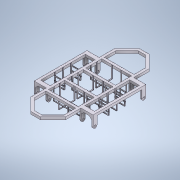
# Autodesk Inventor part: Rahmen_neu
Saved by Autodesk Inventor 2020 (Build 240168000, 168)
## iProperties
Created: 2020-04-28
Part Number: Rahmen_neu
Material: Aluminum 6061, geschweißt
Document SubType Name: Modeling
Designer: Chris
Density: 2.7 g/cm^3
Appearance: Schweißnaht - Aluminum
Mass: 36293.4 g
Surface Area: 46389.4 cm^2
Volume: 13442 cm^3
Author: Chris
Autodesk Inventor part; units mm, degrees
ref_plane "YZ Plane" through (0, 0, 0) normal (1, 0, 0) x (0, 1, 0)
ref_plane "XZ Plane" through (0, 0, 0) normal (0, 1, 0) x (-1, 0, 0)
ref_plane "XY Plane" through (0, 0, 0) normal (0, 0, 1) x (1, 0, 0)
sketch "Skizze1" plane through (0, 0, 0) normal (0, 1, 0) x (-1, 0, 0)
  line L0 (0, 0) -> (590, 0)
  line L1 (590, 0) -> (590, -1060)
  line L2 (590, -1060) -> (0, -1060)
  line L3 (0, -1060) -> (0, 0)
  line L4 (0, 0) -> (-50, 0)
  line L5 (-50, 0) -> (-50, 50)
  line L6 (-50, 50) -> (0, 50)
  line L7 (0, 50) -> (0, 0)
  line L8 (-50, 50) -> (640, 50)
  line L9 (640, 50) -> (640, -1110)
  line L10 (640, -1110) -> (-50, -1110)
  line L11 (-50, -1110) -> (-50, 50)
  line L12 (590, 0) -> (590, -320) construction
  line L13 (590, -320) -> (590, -370) construction
  line L14 (590, -370) -> (590, -690) construction
  line L15 (590, -690) -> (590, -740) construction
  line L16 (590, -740) -> (590, -1060) construction
  line L17 (590, -320) -> (0, -320)
  line L18 (590, -370) -> (0, -370)
  line L19 (590, -690) -> (0, -690)
  line L20 (590, -740) -> (0, -740)
  dimension "d0" = 590
  dimension "d1" = 1060
  dimension "d3" = 50
  dimension "d4" = 50
  dimension "d5" = 690
  dimension "d6" = 1160
  dimension "d38" = 320
  dimension "d39" = 50
  dimension "d40" = 320
  dimension "d41" = 50
  dimension "d42" = 320
  constraints: 42 end point, 8 point on line, 7 perpendicular, 6 parallel, 3 horizontal, 1 collinear
  measures "d0" distance of L1.end L2.end
  measures "d1" distance of L0.end L1.end
  measures "d3" distance of L5.end L6.end
  measures "d4" distance of L4.end L5.end
  measures "d5" distance of L9.end L10.end
  measures "d6" distance of L8.end L9.end
  measures "d38" distance of L0.end L12.end
  measures "d39" distance of L12.end L13.end
  measures "d40" distance of L13.end L14.end
  measures "d41" distance of L14.end L15.end
  measures "d42" distance of L15.end L1.end
extrude "Extrusion1" add sketch "Skizze1" along normal blind 50 contours L7 L8 L9 L10 L11 L4 | L4 L5 L6 L7 | L17 L1 L18 L3 | L19 L1 L20 L3
sketch "Skizze2" plane through (0, 50, 0) normal (0, 1, 0) x (1, 0, 0)
  line L0 (-640, -50) -> (50, -50) projected
  line L1 (-640, -50) -> (-380, -50) construction
  line L2 (50, -300) -> (50, -50)
  line L3 (50, -300) -> (-200, -550)
  line L4 (50, -300) -> (403.5534, -300) construction
  line L5 (-220.7107, -500) -> (0.0003, -279.289)
  line L6 (0.0003, -279.289) -> (0.0003, -50)
  line L7 (-630, 530) -> (45, 530) construction
  line L8 (-640, -50) -> (-640, -550) construction
  line L9 (-640, -50) -> (-140, -50) construction
  line L10 (-640, -50) -> (-640, -300)
  line L11 (-640, -300) -> (-390, -550)
  line L12 (-390, -550) -> (-200, -550)
  line L13 (-515, -425) -> (-479.6447, -389.6447) construction
  line L14 (-640, -50) -> (50, -50) projected
  line L15 (-590, -50) -> (-590, -279.2893)
  line L16 (-590, -279.2893) -> (-369.2893, -500)
  line L17 (-369.2893, -500) -> (-220.7107, -500)
  line L18 (-640, -50) -> (-590, -50)
  line L19 (0.0003, -50) -> (50, -50)
  line L20 (-640, 1110) -> (50, 1110)
  line L21 (-640, 1110) -> (-380, 1110) construction
  line L22 (50, 1360) -> (50, 1110)
  line L23 (50, 1360) -> (-200, 1610)
  line L24 (50, 1360) -> (403.5534, 1360) construction
  line L25 (-220.7107, 1560) -> (0.0003, 1339.289)
  line L26 (0.0003, 1339.289) -> (0.0003, 1110)
  line L27 (-640, 1110) -> (-640, 1610) construction
  line L28 (-640, 1110) -> (-140, 1110) construction
  line L29 (-640, 1110) -> (-640, 1360)
  line L30 (-640, 1360) -> (-390, 1610)
  line L31 (-390, 1610) -> (-200, 1610)
  line L32 (-515, 1485) -> (-479.6447, 1449.6447) construction
  line L33 (-640, 1110) -> (50, 1110)
  line L34 (-590, 1110) -> (-590, 1339.2893)
  line L35 (-590, 1339.2893) -> (-369.2893, 1560)
  line L36 (-369.2893, 1560) -> (-220.7107, 1560)
  line L37 (-640, 1110) -> (-590, 1110)
  line L38 (0.0003, 1110) -> (50, 1110)
  point P0 (0, 0)
  point P1 (-640, 1110)
  point P2 (50, 1110)
  point P3 (0, 1060)
  dimension "d13" = 250
  dimension "d14" = 90
  dimension "d28" = 135
  dimension "d32" = 50
  dimension "d33" = 220.711
  dimension "d81" = 500
  dimension "d82" = 90
  dimension "d83" = 250
  dimension "d84" = 135
  dimension "d87" = 50
  dimension "d88" = 50
  dimension "d89" = 50
  constraints: 74 end point, 21 symmetric about line, 5 horizontal, 4 point on line, 3 midpoint, 3 perpendicular, 2 equal length, 1 collinear, 1 vertical
  measures "d13" distance of L2.start L0.end
  measures "d14" angle of L2 L0
  measures "d28" angle of L3 L4
  measures "d32" distance between parallel lines of L3 L5
  measures "d33" horizontal distance of L5.start L5.end
  measures "d81" distance of L0.start L8.end
  measures "d82" angle of L8 L9
  measures "d83" distance of L0.start L10.end
  measures "d84" angle of L11 L10
  measures "d87" distance of L13.start L13.end
  measures "d88" distance between parallel lines of L12 L17
  measures "d89" distance between parallel lines of L15 L8
extrude "Extrusion2" add sketch "Skizze2" against normal blind 50 contours L0 L15 L16 L17 L5 L6 L2 L3 L12 L11 L10 | L29 L30 L31 L23 L22 L20 L26 L25 L36 L35 L34
sketch "Skizze3" plane through (0, 50, 0) normal (0, 1, 0) x (1, 0, 0)
  line L0 (-590, 370) -> (-590, 690) construction
  line L1 (-634.8333, 530) -> (-634.8333, 1015) construction
  line L2 (-640, 1360) -> (-640, -300) construction
  line L3 (-200, -550) -> (-380, -550) construction
  line L4 (-380, 1610) -> (-200, 1610) construction
  line L5 (-640, 530) -> (-640, 45) construction
  line L6 (-640, 45) -> (-880, 45)
  line L7 (-880, 45) -> (-880, 85)
  line L8 (-880, 85) -> (-640, 85)
  line L9 (-640, 85) -> (-640, 45)
  line L10 (-640, 45) -> (-880, 45)
  line L11 (-880, 45) -> (-880, 5)
  line L12 (-880, 5) -> (-640, 5)
  line L13 (-640, 5) -> (-640, 45)
  line L14 (50, -300) -> (50, 1360) projected
  line L15 (50, 530) -> (-640, 530)
  line L16 (-390, -550) -> (-200, -550) projected
  line L17 (-295, -550) -> (-295, 1610)
  line L18 (-390, 1610) -> (-200, 1610) projected
  line L19 (50, 45) -> (290, 45)
  line L20 (290, 45) -> (290, 85)
  line L21 (290, 85) -> (50, 85)
  line L22 (50, 85) -> (50, 45)
  line L23 (50, 45) -> (290, 45)
  line L24 (290, 45) -> (290, 5)
  line L25 (290, 5) -> (50, 5)
  line L26 (50, 5) -> (50, 45)
  line L27 (-640, 1015) -> (-880, 1015)
  line L28 (-880, 1015) -> (-880, 975)
  line L29 (-880, 975) -> (-640, 975)
  line L30 (-640, 975) -> (-640, 1015)
  line L31 (-640, 1015) -> (-880, 1015)
  line L32 (-880, 1015) -> (-880, 1055)
  line L33 (-880, 1055) -> (-640, 1055)
  line L34 (-640, 1055) -> (-640, 1015)
  line L35 (50, 975) -> (50, 1015)
  line L36 (50, 1055) -> (50, 1015)
  line L37 (290, 1015) -> (290, 975)
  line L38 (290, 975) -> (50, 975)
  line L39 (290, 1055) -> (50, 1055)
  line L40 (50, 1015) -> (290, 1015)
  line L41 (290, 1015) -> (290, 1055)
  line L42 (50, 1015) -> (290, 1015)
  point P0 (0, 0)
  point P1 (-640, 1330)
  point P2 (-630, -300)
  point P3 (-640, -50)
  point P4 (-640, -300)
  point P5 (50, 1110)
  point P6 (50, -50)
  point P7 (0, 1060)
  point P8 (-640, 1110)
  point P9 (50, 1110)
  dimension "d45" = 485
  dimension "d51" = 240
  dimension "d52" = 40
  dimension "d53" = 40
  dimension "d62" = 485
  dimension "d91" = 90
  constraints: 72 end point, 25 symmetric about line, 4 parallel, 4 point on line, 3 midpoint, 3 perpendicular, 2 horizontal, 1 vertical, 3 other
  measures "d45" distance of L1.start L1.end
  measures "d51" distance of L7.end L8.end
  measures "d52" distance of L6.end L7.end
  measures "d53" distance of L11.end L10.end
  measures "d62" distance from line of L5.start L6
  measures "d91" angle of L17 L15
extrude "Extrusion3" add sketch "Skizze3" against normal blind 50
sketch "Skizze6" plane through (0, 50, 0) normal (0, 1, 0) x (1, 0, 0)
  line L0 (-880, 975) -> (-645, 975) projected
  line L1 (-640, 85) -> (-880, 85) projected
  line L2 (-880, 975) -> (-830, 975)
  line L3 (-830, 975) -> (-830, 85)
  line L4 (-830, 85) -> (-880, 85)
  line L5 (-880, 85) -> (-880, 975)
  line L6 (50, 85) -> (290, 85) projected
  line L7 (290, 975) -> (55, 975) projected
  line L8 (290, 85) -> (240, 85)
  line L9 (240, 85) -> (240, 975)
  line L10 (240, 975) -> (290, 975)
  line L11 (290, 975) -> (290, 85)
  point P0 (-640, 975)
  point P1 (-880, 85)
  point P2 (50, 975)
  point P3 (290, 975)
  point P4 (240, 85)
  dimension "d69" = 50
  dimension "d92" = 50
  constraints: 16 end point, 4 parallel, 2 horizontal, 2 perpendicular, 2 point on line
  measures "d69" distance of L3.end L4.end
  measures "d92" distance of L9.end L10.end
extrude "Extrusion5" add sketch "Skizze6" against normal blind 50
shell "Wandung3" thickness 5 removed faces 0
sketch "Skizze5" plane through (0, 0, 0) normal (0, -1, 0) x (1, 0, 0)
  line L0 (-202.0711, -1605) -> (-387.9289, -1605) construction
  line L1 (-295, -1605) -> (-295, 545) construction
  line L2 (-202.0711, 545) -> (-387.9289, 545) construction
  line L3 (290, -1055) -> (290, -5) projected
  line L4 (290, -5) -> (265, -5)
  line L5 (265, -5) -> (265, -85)
  line L6 (265, -85) -> (290, -85)
  line L7 (290, -85) -> (290, -5)
  line L8 (50, -5) -> (290, -5) construction
  line L9 (265, -5) -> (50, -5) construction
  line L10 (265, -5) -> (480, -5) construction
  line L11 (269.9902, -1052.9524) -> (484.9805, -1050.9049) construction
  line L12 (-880, -1055) -> (-880, -5)
  line L13 (-855, -5) -> (-1070, -5) construction
  line L14 (-859.9902, -1052.9524) -> (-1074.9805, -1050.9049) construction
  line L15 (265, -5) -> (55, -5) construction
  line L16 (290, -5) -> (50, -5) construction
  line L17 (55, -5) -> (30, -5)
  line L18 (30, -5) -> (30, -85)
  line L19 (30, -85) -> (55, -85)
  line L20 (55, -85) -> (55, -5)
  line L21 (-880, -5) -> (-855, -5)
  line L22 (-855, -5) -> (-855, -85)
  line L23 (-855, -85) -> (-880, -85)
  line L24 (-880, -85) -> (-880, -5)
  line L25 (-645, -5) -> (-620, -5)
  line L26 (-620, -5) -> (-620, -85)
  line L27 (-620, -85) -> (-645, -85)
  line L28 (-645, -85) -> (-645, -5)
  line L29 (-880, -5) -> (-880, -1055) projected
  line L30 (-880, -530) -> (290, -530)
  line L31 (290, -1055) -> (265, -1055)
  line L32 (265, -1055) -> (265, -975)
  line L33 (265, -975) -> (290, -975)
  line L34 (290, -975) -> (290, -1055)
  line L35 (55, -1055) -> (30, -1055)
  line L36 (30, -1055) -> (30, -975)
  line L37 (30, -975) -> (55, -975)
  line L38 (55, -975) -> (55, -1055)
  line L39 (-620, -975) -> (-645, -975)
  line L40 (-620, -1055) -> (-620, -975)
  line L41 (-645, -975) -> (-645, -1055)
  line L42 (-645, -1055) -> (-620, -1055)
  line L43 (-880, -1055) -> (-855, -1055)
  line L44 (-855, -975) -> (-880, -975)
  line L45 (-855, -1055) -> (-855, -975)
  line L46 (-880, -975) -> (-880, -1055)
  point P0 (290, -85)
  point P1 (-640, -5)
  point P2 (50, -1055)
  point P3 (-640, -1055)
  dimension "d93" = 25
  dimension "d94" = 80
  dimension "d96" = 180
  dimension "d155" = 210
  dimension "d156" = 25
  constraints: 82 end point, 29 symmetric about line, 4 midpoint, 4 parallel, 3 horizontal, 2 collinear, 2 perpendicular, 1 point on line
  measures "d93" distance of L6.end L5.end
  measures "d94" distance of L5.end L4.end
  measures "d96" angle of L10 L9
  measures "d155" distance of L4.end L15.end
  measures "d156" distance of L19.end L18.end
extrude "Extrusion9" add sketch "Skizze5" along normal blind 200
sketch "Skizze10" plane through (290, 50, -5) normal (1, 0, 0) x (0, 0, -1)
  line L0 (970, -250) -> (1050, -250) construction
  line L1 (970, -250) -> (1010, -250) construction
  line L2 (1010, -250) -> (1010, -210) construction
  line L3 (1010, -210) -> (970, -210) construction
  line L4 (970, -210) -> (970, -250) construction
  circle A0 centre (1010, -210) radius 20
  line L5 (0, -250) -> (40, -250) construction
  line L6 (40, -250) -> (40, -210) construction
  line L7 (40, -210) -> (0, -210) construction
  line L8 (0, -210) -> (0, -250) construction
  circle A1 centre (40, -210) radius 20
  dimension "d157" = 40
  dimension "d158" = 40
  dimension "d159" = 40
  dimension "d214" = 40
  dimension "d215" = 40
  dimension "d216" = 40
  constraints: 16 end point, 4 parallel, 2 centre point, 2 coincident, 2 horizontal, 2 perpendicular
  measures "d157" distance of L3.end L2.end
  measures "d158" distance of L2.end L1.end
  measures "d159" diameter of A0
  measures "d214" distance of L7.end L6.end
  measures "d215" distance of L6.end L5.end
  measures "d216" diameter of A1
extrude "Extrusion10" cut sketch "Skizze10" against normal blind 1500
fillet "Rundung3" radius 40 16 edges at (277.5, -200, -5) (277.5, -200, -85) (42.5, -200, -5) (42.5, -200, -85) (277.5, -200, -975) (277.5, -200, -1055) (42.5, -200, -975) (42.5, -200, -1055) (-632.5, -200, -5) (-632.5, -200, -85) (-867.5, -200, -5) (-867.5, -200, -85) (-632.5, -200, -975) (-632.5, -200, -1055) (-867.5, -200, -975) (-867.5, -200, -1055)
sketch "Skizze11" plane through (0, 50, 0) normal (0, 1, 0) x (1, 0, 0)
  line L0 (0, 0) -> (-200, 0) construction
  line L1 (0, 0) -> (-590, 0) construction
  line L2 (-590, 0) -> (-390, 0) construction
  line L3 (-590, 320) -> (0, 320) construction
  line L4 (0, 320) -> (0, 220) construction
  line L5 (0, 320) -> (0, 0) construction
  line L6 (0, 0) -> (0, 100) construction
  line L7 (-200, 0) -> (-190, 0) construction
  line L8 (-390, 0) -> (-400, 0) construction
  line L9 (0, 100) -> (0, 90) construction
  line L10 (0, 220) -> (0, 230) construction
  line L11 (0, 90) -> (-5, 90)
  line L12 (-5, 90) -> (-5, 110)
  line L13 (-5, 110) -> (0, 110)
  line L14 (0, 110) -> (0, 90)
  line L15 (0, 220) -> (-5, 220)
  line L16 (-5, 220) -> (-5, 240)
  line L17 (-5, 240) -> (0, 240)
  line L18 (0, 240) -> (0, 220)
  line L19 (-190, 0) -> (-210, 0)
  line L20 (-210, 0) -> (-210, 5)
  line L21 (-210, 5) -> (-190, 5)
  line L22 (-190, 5) -> (-190, 0)
  line L23 (-400, 0) -> (-380, 0)
  line L24 (-380, 0) -> (-380, 5)
  line L25 (-380, 5) -> (-400, 5)
  line L26 (-400, 5) -> (-400, 0)
  line L27 (5, 325) -> (5, -5) projected
  line L28 (5, 160) -> (-590, 160)
  line L29 (-590, 0) -> (-590, 320) projected
  line L30 (-295, 0) -> (-295, 320)
  line L31 (-590, 100) -> (-590, 90) construction
  line L32 (-590, 220) -> (-590, 230) construction
  line L33 (-590, 90) -> (-585, 90)
  line L34 (-585, 90) -> (-585, 110)
  line L35 (-585, 110) -> (-590, 110)
  line L36 (-590, 110) -> (-590, 90)
  line L37 (-590, 220) -> (-585, 220)
  line L38 (-585, 220) -> (-585, 240)
  line L39 (-585, 240) -> (-590, 240)
  line L40 (-590, 240) -> (-590, 220)
  line L41 (-200, 320) -> (-190, 320) construction
  line L42 (-390, 320) -> (-400, 320) construction
  line L43 (-190, 320) -> (-210, 320)
  line L44 (-210, 320) -> (-210, 315)
  line L45 (-210, 315) -> (-190, 315)
  line L46 (-190, 315) -> (-190, 320)
  line L47 (-400, 320) -> (-380, 320)
  line L48 (-380, 320) -> (-380, 315)
  line L49 (-380, 315) -> (-400, 315)
  line L50 (-400, 315) -> (-400, 320)
  line L51 (0, 690) -> (0, 370) projected
  line L52 (0, 530) -> (-590, 530)
  line L53 (-590, 370) -> (-590, 690) projected
  line L54 (0, 370) -> (-590, 370) projected
  line L55 (-295, 370) -> (-295, 690)
  line L56 (-590, 690) -> (0, 690) projected
  line L57 (0, 370) -> (-190, 370) construction
  line L58 (-590, 370) -> (-400, 370) construction
  line L59 (0, 370) -> (0, 460) construction
  line L60 (0, 690) -> (0, 600) construction
  line L61 (0, 600) -> (-5, 600)
  line L62 (-5, 600) -> (-5, 580)
  line L63 (-5, 580) -> (0, 580)
  line L64 (0, 580) -> (0, 600)
  line L65 (0, 460) -> (-5, 460)
  line L66 (-5, 460) -> (-5, 480)
  line L67 (-5, 480) -> (0, 480)
  line L68 (0, 480) -> (0, 460)
  line L69 (-190, 370) -> (-210, 370)
  line L70 (-210, 370) -> (-210, 375)
  line L71 (-210, 375) -> (-190, 375)
  line L72 (-190, 375) -> (-190, 370)
  line L73 (-400, 370) -> (-380, 370)
  line L74 (-380, 370) -> (-380, 375)
  line L75 (-380, 375) -> (-400, 375)
  line L76 (-400, 375) -> (-400, 370)
  line L77 (-590, 600) -> (-585, 600)
  line L78 (-585, 600) -> (-585, 580)
  line L79 (-585, 580) -> (-590, 580)
  line L80 (-590, 580) -> (-590, 600)
  line L81 (-590, 460) -> (-585, 460)
  line L82 (-585, 460) -> (-585, 480)
  line L83 (-585, 480) -> (-590, 480)
  line L84 (-590, 480) -> (-590, 460)
  line L85 (-190, 690) -> (-210, 690)
  line L86 (-210, 690) -> (-210, 685)
  line L87 (-210, 685) -> (-190, 685)
  line L88 (-190, 685) -> (-190, 690)
  line L89 (-400, 690) -> (-380, 690)
  line L90 (-380, 690) -> (-380, 685)
  line L91 (-380, 685) -> (-400, 685)
  line L92 (-400, 685) -> (-400, 690)
  line L93 (0, 690) -> (0, 715) construction
  line L94 (0, 715) -> (-590, 715) construction
  line L95 (0, 740) -> (-590, 740) construction
  line L96 (-295, 740) -> (-295, 1060) construction
  line L97 (-590, 1060) -> (0, 1060) construction
  line L98 (0, 1060) -> (0, 740) construction
  line L99 (0, 900) -> (-590, 900) construction
  line L100 (-590, 740) -> (-590, 1060) construction
  line L101 (-400, 745) -> (-400, 740)
  line L102 (-400, 740) -> (-380, 740)
  line L103 (-380, 745) -> (-400, 745)
  line L104 (-380, 740) -> (-380, 745)
  line L105 (-210, 740) -> (-210, 745)
  line L106 (-210, 745) -> (-190, 745)
  line L107 (-190, 740) -> (-210, 740)
  line L108 (-190, 745) -> (-190, 740)
  line L109 (-210, 1060) -> (-210, 1055)
  line L110 (-210, 1055) -> (-190, 1055)
  line L111 (-190, 1055) -> (-190, 1060)
  line L112 (-190, 1060) -> (-210, 1060)
  line L113 (-380, 1060) -> (-380, 1055)
  line L114 (-400, 1060) -> (-380, 1060)
  line L115 (-380, 1055) -> (-400, 1055)
  line L116 (-400, 1055) -> (-400, 1060)
  line L117 (0, 830) -> (-5, 830)
  line L118 (-5, 830) -> (-5, 850)
  line L119 (-5, 850) -> (0, 850)
  line L120 (0, 850) -> (0, 830)
  line L121 (0, 970) -> (-5, 970)
  line L122 (-5, 970) -> (-5, 950)
  line L123 (-5, 950) -> (0, 950)
  line L124 (0, 950) -> (0, 970)
  line L125 (-590, 970) -> (-585, 970)
  line L126 (-585, 970) -> (-585, 950)
  line L127 (-585, 950) -> (-590, 950)
  line L128 (-585, 830) -> (-585, 850)
  line L129 (-590, 830) -> (-585, 830)
  line L130 (-590, 850) -> (-590, 830)
  line L131 (-585, 850) -> (-590, 850)
  line L132 (-590, 950) -> (-590, 970)
  point P0 (-595, 160)
  dimension "d112" = 200
  dimension "d115" = 200
  dimension "d116" = 100
  dimension "d117" = 100
  dimension "d118" = 10
  dimension "d119" = 10
  dimension "d120" = 10
  dimension "d121" = 10
  dimension "d122" = 5
  dimension "d123" = 20
  dimension "d124" = 5
  dimension "d125" = 20
  dimension "d126" = 20
  dimension "d127" = 5
  dimension "d128" = 20
  dimension "d129" = 5
  dimension "d130" = 190
  dimension "d131" = 190
  dimension "d132" = 90
  dimension "d133" = 90
  dimension "d134" = 5
  dimension "d135" = 20
  dimension "d136" = 5
  dimension "d137" = 20
  dimension "d138" = 20
  dimension "d139" = 5
  dimension "d140" = 20
  dimension "d141" = 5
  dimension "d142" = 25
  dimension "d143" = 590
  dimension "d144" = 90
  constraints: 240 end point, 69 symmetric about line, 16 parallel, 12 midpoint, 11 point on line, 9 perpendicular, 8 horizontal, 1 vertical
  measures "d112" distance of L0.start L0.end
  measures "d115" distance of L1.end L2.end
  measures "d116" distance of L3.end L4.end
  measures "d117" distance of L0.start L6.end
  measures "d118" distance of L0.end L7.end
  measures "d119" distance of L2.end L8.end
  measures "d120" distance of L6.end L9.end
  measures "d121" distance of L4.end L10.end
  measures "d122" distance of L12.end L13.end
  measures "d123" distance of L11.end L12.end
  measures "d124" distance of L16.end L17.end
  measures "d125" distance of L15.end L16.end
  measures "d126" distance of L20.end L21.end
  measures "d127" distance of L19.end L20.end
  measures "d128" distance of L25.end L24.end
  measures "d129" distance of L24.end L23.end
  measures "d130" distance of L51.end L57.end
  measures "d131" distance of L53.start L58.end
  measures "d132" distance of L51.end L59.end
  measures "d133" distance of L51.start L60.end
  measures "d134" distance of L63.end L62.end
  measures "d135" distance of L62.end L61.end
  measures "d136" distance of L66.end L67.end
  measures "d137" distance of L65.end L66.end
  measures "d138" distance of L70.end L71.end
  measures "d139" distance of L69.end L70.end
  measures "d140" distance of L75.end L74.end
  measures "d141" distance of L74.end L73.end
  measures "d142" distance of L51.start L93.end
  measures "d143" distance of L93.end L94.end
  measures "d144" angle of L94 L93
extrude "Extrusion11" add sketch "Skizze11" against normal blind 240 contours L11 L12 L13 L14 | L15 L16 L17 L18 | L19 L20 L21 L22 | L26 L25 L24 L23 | L29 L35 L34 L33 | L29 L39 L38 L37 | L46 L45 L44 L43 | L47 L48 L49 L50 | L51 L63 L62 L61 | L88 L87 L86 L56 | L51 L65 L66 L67 | L90 L91 L92 L56 | L83 L82 L81 L53 | L53 L77 L78 L79 | L70 L71 L72 L54 | L54 L76 L75 L74 | L103 L104 L102 L101 | L105 L106 L108 L107 | L112 L111 L110 L109 | L113 L115 L116 L114 | L117 L118 L119 L120 | L124 L123 L122 L121 | L125 L126 L127 L132 | L129 L130 L131 L128
sketch "Skizze12" plane through (-590, 50, -90) normal (0, 0, 1) x (1, 0, 0)
  line L0 (0, -240) -> (5, -240) projected
  line L1 (5, 0) -> (5, -240) projected
  line L2 (0, -240) -> (5, -240)
  line L3 (5, -240) -> (5, -235)
  line L4 (5, -235) -> (0, -235)
  line L5 (0, -235) -> (0, -240)
  line L6 (590, -240) -> (585, -240) projected
  line L7 (590, -50) -> (590, -240) projected
  line L8 (585, -240) -> (590, -240)
  line L9 (590, -240) -> (590, -235)
  line L10 (590, -235) -> (585, -235)
  line L11 (585, -235) -> (585, -240)
  dimension "d147" = 5
  dimension "d148" = 5
  constraints: 16 end point, 4 parallel, 2 horizontal, 2 perpendicular, 2 point on line
  measures "d147" distance of L3.end L2.end
  measures "d148" distance of L9.end L8.end
extrude "Extrusion12" cut sketch "Skizze12" against normal blind 2000
sketch "Skizze13" plane through (-590, -185, -950) normal (0, -1, 0) x (1, 0, 0)
  line L0 (590, -20) -> (590, 0) projected
  line L1 (0, 0) -> (590, 0)
  line L2 (590, 0) -> (590, -20)
  line L3 (590, -20) -> (0, -20)
  line L4 (0, -20) -> (0, 0)
  line L5 (0, 120) -> (0, 100) projected
  line L6 (590, 100) -> (585, 100) projected
  line L7 (0, 120) -> (590, 120)
  line L8 (590, 120) -> (590, 100)
  line L9 (590, 100) -> (0, 100)
  line L10 (0, 100) -> (0, 120)
  line L11 (0, 370) -> (5, 370) projected
  line L12 (590, 350) -> (590, 370) projected
  line L13 (0, 370) -> (590, 370)
  line L14 (590, 370) -> (590, 350)
  line L15 (590, 350) -> (0, 350)
  line L16 (0, 350) -> (0, 370)
  line L17 (590, 470) -> (585, 470) projected
  line L18 (0, 490) -> (590, 490)
  line L19 (590, 490) -> (590, 470)
  line L20 (590, 470) -> (0, 470)
  line L21 (0, 470) -> (0, 490)
  line L22 (0, 730) -> (0, 710) projected
  line L23 (590, 730) -> (590, 710) projected
  line L24 (0, 730) -> (590, 730)
  line L25 (590, 730) -> (590, 710)
  line L26 (590, 710) -> (0, 710)
  line L27 (0, 710) -> (0, 730)
  line L28 (0, 860) -> (0, 840) projected
  line L29 (590, 860) -> (590, 840) projected
  line L30 (0, 860) -> (590, 860)
  line L31 (590, 860) -> (590, 840)
  line L32 (590, 840) -> (0, 840)
  line L33 (0, 840) -> (0, 860)
  point P0 (590, 950)
  point P1 (590, 0)
  point P2 (0, 100)
  point P3 (585, 100)
  point P4 (590, 370)
  point P5 (5, 370)
  point P6 (585, 470)
  point P7 (590, 730)
  point P8 (0, 710)
  point P9 (0, 840)
  point P10 (590, 860)
  constraints: 48 end point, 12 parallel, 6 horizontal, 6 perpendicular
extrude "Extrusion13" add sketch "Skizze13" along normal blind 5
sketch "Skizze14" plane through (0, -190, 0) normal (0, -1, 0) x (1, 0, 0)
  line L0 (-400, 0) -> (-590, 0) projected
  line L1 (-380, -320) -> (-380, -315) projected
  line L2 (-400, 0) -> (-380, 0)
  line L3 (-380, 0) -> (-380, -320)
  line L4 (-380, -320) -> (-400, -320)
  line L5 (-400, -320) -> (-400, 0)
  line L6 (-190, -320) -> (0, -320) projected
  line L7 (-210, 0) -> (-380, 0) projected
  line L8 (-190, -320) -> (-210, -320)
  line L9 (-210, -320) -> (-210, 0)
  line L10 (-210, 0) -> (-190, 0)
  line L11 (-190, 0) -> (-190, -320)
  line L12 (-380, -370) -> (-400, -370) projected
  line L13 (-400, -690) -> (-380, -690) projected
  line L14 (-400, -370) -> (-380, -370)
  line L15 (-380, -370) -> (-380, -690)
  line L16 (-380, -690) -> (-400, -690)
  line L17 (-400, -690) -> (-400, -370)
  line L18 (-210, -690) -> (-190, -690) projected
  line L19 (-210, -370) -> (-380, -370) projected
  line L20 (-190, -690) -> (-210, -690)
  line L21 (-210, -690) -> (-210, -370)
  line L22 (-210, -370) -> (-190, -370)
  line L23 (-190, -370) -> (-190, -690)
  line L24 (-400, -740) -> (-400, -745) projected
  line L25 (-380, -1060) -> (-400, -1060)
  line L26 (-400, -1060) -> (-400, -740)
  line L27 (-400, -740) -> (-380, -740)
  line L28 (-380, -740) -> (-380, -1060)
  line L29 (-210, -745) -> (-210, -740) projected
  line L30 (-190, -1060) -> (-210, -1060)
  line L31 (-210, -1060) -> (-210, -740)
  line L32 (-210, -740) -> (-190, -740)
  line L33 (-190, -740) -> (-190, -1060)
  point P0 (0, 0)
  constraints: 48 end point, 12 parallel, 6 horizontal, 6 perpendicular
extrude "Extrusion14" add sketch "Skizze14" along normal blind 5
sketch "Skizze15" plane through (0, 50, 0) normal (0, 1, 0) x (1, 0, 0)
  line L0 (240, 85) -> (50, 85) construction
  line L1 (50, 85) -> (50, 360) construction
  line L2 (50, 85) -> (325, 85) construction
  line L3 (50, 360) -> (55, 360)
  line L4 (55, 360) -> (55, 380)
  line L5 (55, 380) -> (50, 380)
  line L6 (50, 380) -> (50, 360)
  line L7 (50, 380) -> (50, 520) construction
  line L8 (45, 80) -> (45, 980) construction
  line L9 (50, 380) -> (190, 380) construction
  line L10 (50, 520) -> (55, 520)
  line L11 (55, 520) -> (55, 540)
  line L12 (55, 540) -> (50, 540)
  line L13 (50, 540) -> (50, 520)
  line L14 (50, 540) -> (50, 680) construction
  line L15 (50, 85) -> (50, 975) construction
  line L16 (50, 680) -> (55, 680)
  line L17 (55, 680) -> (55, 700)
  line L18 (55, 700) -> (50, 700)
  line L19 (50, 700) -> (50, 680)
  line L20 (240, 975) -> (240, 85) construction
  line L21 (240, 85) -> (50, 85) construction
  line L22 (145, 85) -> (145, 975) construction
  line L23 (50, 975) -> (240, 975) construction
  line L24 (145, 85) -> (1035, 85) construction
  line L25 (240, 360) -> (235, 360)
  line L26 (235, 360) -> (235, 380)
  line L27 (235, 380) -> (240, 380)
  line L28 (240, 380) -> (240, 360)
  line L29 (240, 520) -> (235, 520)
  line L30 (235, 520) -> (235, 540)
  line L31 (235, 540) -> (240, 540)
  line L32 (240, 540) -> (240, 520)
  line L33 (240, 680) -> (235, 680)
  line L34 (235, 680) -> (235, 700)
  line L35 (235, 700) -> (240, 700)
  line L36 (240, 700) -> (240, 680)
  point P0 (0, 0)
  dimension "d160" = 275
  dimension "d161" = 90
  dimension "d162" = 5
  dimension "d163" = 20
  dimension "d164" = 140
  dimension "d165" = 90
  dimension "d166" = 5
  dimension "d167" = 20
  dimension "d168" = 140
  dimension "d169" = 5
  dimension "d170" = 20
  dimension "d171" = 90
  constraints: 64 end point, 12 symmetric about line, 7 parallel, 6 horizontal, 6 perpendicular, 2 midpoint, 1 collinear, 1 point on line, 1 vertical
  measures "d160" distance of L0.end L1.end
  measures "d161" angle of L2 L1
  measures "d162" distance of L5.end L4.end
  measures "d163" distance of L4.end L3.end
  measures "d164" distance of L5.end L7.end
  measures "d165" angle of L9 L7
  measures "d166" distance of L12.end L11.end
  measures "d167" distance of L11.end L10.end
  measures "d168" distance of L12.end L14.end
  measures "d169" distance of L18.end L17.end
  measures "d170" distance of L17.end L16.end
  measures "d171" angle of L24 L22
extrude "Extrusion15" add sketch "Skizze15" against normal blind 210
sketch "Skizze16" plane through (0, -160, 0) normal (0, -1, 0) x (1, 0, 0)
  line L0 (50, -360) -> (55, -360) projected
  line L1 (240, -380) -> (235, -380) projected
  line L2 (50, -360) -> (240, -360)
  line L3 (240, -360) -> (240, -380)
  line L4 (240, -380) -> (50, -380)
  line L5 (50, -380) -> (50, -360)
  line L6 (55, -520) -> (50, -520) projected
  line L7 (240, -540) -> (240, -520) projected
  line L8 (50, -520) -> (240, -520)
  line L9 (240, -520) -> (240, -540)
  line L10 (240, -540) -> (50, -540)
  line L11 (50, -540) -> (50, -520)
  line L12 (50, -700) -> (50, -680) projected
  line L13 (235, -700) -> (240, -700) projected
  line L14 (50, -680) -> (240, -680)
  line L15 (240, -680) -> (240, -700)
  line L16 (240, -700) -> (50, -700)
  line L17 (50, -700) -> (50, -680)
  point P0 (0, 0)
  constraints: 24 end point, 6 parallel, 3 horizontal, 3 perpendicular
extrude "Extrusion16" add sketch "Skizze16" along normal blind 5
sketch "Skizze17" plane through (50, 0, -360) normal (0, 0, 1) x (1, 0, 0)
  line L0 (185, -160) -> (5, -160) construction
  line L1 (185, -160) -> (185, -110) construction
  line L2 (190, 0) -> (190, -165) projected
  line L3 (0, 0) -> (0, -165) projected
  line L4 (190, -110) -> (0, -110)
  line L5 (0, -110) -> (0, -90)
  line L6 (0, -90) -> (190, -90)
  line L7 (190, -90) -> (190, -110)
  line L8 (190, 0) -> (0, 0)
  line L9 (0, 0) -> (0, -20)
  line L10 (0, -20) -> (190, -20)
  line L11 (190, -20) -> (190, 0)
  point P0 (-50, 0)
  dimension "d176" = 50
  dimension "d177" = 20
  dimension "d178" = 190
  dimension "d179" = 20
  constraints: 18 end point, 4 parallel, 2 horizontal, 2 perpendicular, 2 point on line, 1 vertical
  measures "d176" distance of L0.start L1.end
  measures "d177" distance of L4.end L5.end
  measures "d178" distance of L10.end L9.end
  measures "d179" distance of L9.end L8.end
extrude "Extrusion17" add sketch "Skizze17" along normal blind 5 contours L2 L10 L3 L8 | L2 L4 L3 L6
sketch "Skizze18" plane through (50, 0, -355) normal (0, 0, 1) x (1, 0, 0)
  line L0 (190, 0) -> (190, -165) projected
  line L1 (190, 0) -> (195, 0)
  line L2 (195, 0) -> (195, -20)
  line L3 (195, -20) -> (190, -20)
  line L4 (190, -20) -> (190, 0)
  line L5 (190, -110) -> (190, -90) projected
  line L6 (190, -90) -> (195, -90)
  line L7 (195, -90) -> (195, -110)
  line L8 (195, -110) -> (190, -110)
  line L9 (190, -110) -> (190, -90)
  line L10 (0, -90) -> (5, -90) projected
  line L11 (0, -90) -> (-5, -90)
  line L12 (-5, -90) -> (-5, -110)
  line L13 (-5, -110) -> (0, -110)
  line L14 (0, -110) -> (0, -90)
  line L15 (0, -20) -> (-5, -20)
  line L16 (-5, -20) -> (-5, 0)
  line L17 (-5, 0) -> (0, 0)
  line L18 (0, 0) -> (0, -20)
  point P0 (-50, 0)
  dimension "d182" = 5
  dimension "d183" = 20
  dimension "d184" = 5
  dimension "d185" = 20
  dimension "d186" = 5
  dimension "d187" = 5
  dimension "d188" = 20
  constraints: 32 end point, 8 parallel, 4 horizontal, 4 perpendicular, 3 point on line
  measures "d182" distance of L2.end L3.end
  measures "d183" distance of L1.end L2.end
  measures "d184" distance of L7.end L8.end
  measures "d185" distance of L6.end L7.end
  measures "d186" distance of L13.end L12.end
  measures "d187" distance of L16.end L17.end
  measures "d188" distance of L15.end L16.end
extrude "Extrusion18" add sketch "Skizze18" against normal blind 25
sketch "Skizze20" plane through (240, 0, -700) normal (0, 0, -1) x (-1, 0, 0)
  line L0 (190, 0) -> (190, -165) projected
  line L1 (190, 0) -> (0, 0)
  line L2 (0, 0) -> (0, -20)
  line L3 (0, -20) -> (190, -20)
  line L4 (190, -20) -> (190, 0)
  line L5 (190, -165) -> (190, -110) construction
  line L6 (190, -110) -> (0, -110)
  line L7 (0, -110) -> (0, -90)
  line L8 (0, -90) -> (190, -90)
  line L9 (190, -90) -> (190, -110)
  point P0 (240, 0)
  dimension "d197" = 190
  dimension "d198" = 20
  dimension "d199" = 55
  dimension "d200" = 190
  dimension "d201" = 20
  constraints: 18 end point, 4 parallel, 2 horizontal, 2 perpendicular, 1 point on line
  measures "d197" distance of L3.end L2.end
  measures "d198" distance of L2.end L1.end
  measures "d199" distance of L0.end L5.end
  measures "d200" distance of L7.end L8.end
  measures "d201" distance of L6.end L7.end
extrude "Extrusion20" add sketch "Skizze20" along normal blind 5
sketch "Skizze21" plane through (240, 0, -705) normal (0, 0, -1) x (-1, 0, 0)
  line L0 (190, 0) -> (195, 0)
  line L1 (195, 0) -> (195, -20)
  line L2 (195, -20) -> (190, -20)
  line L3 (190, -20) -> (190, 0)
  line L4 (190, -110) -> (195, -110)
  line L5 (195, -110) -> (195, -90)
  line L6 (195, -90) -> (190, -90)
  line L7 (190, -90) -> (190, -110)
  line L8 (0, -110) -> (190, -110) projected
  line L9 (0, -110) -> (-5, -110)
  line L10 (-5, -110) -> (-5, -90)
  line L11 (-5, -90) -> (0, -90)
  line L12 (0, -90) -> (0, -110)
  line L13 (0, 0) -> (-5, 0)
  line L14 (-5, 0) -> (-5, -20)
  line L15 (-5, -20) -> (0, -20)
  line L16 (0, -20) -> (0, 0)
  point P0 (240, 0)
  dimension "d204" = 5
  dimension "d205" = 20
  dimension "d206" = 5
  dimension "d207" = 20
  dimension "d208" = 5
  dimension "d209" = 20
  dimension "d210" = 5
  dimension "d211" = 20
  constraints: 32 end point, 8 parallel, 4 horizontal, 4 perpendicular, 1 point on line
  measures "d204" distance of L1.end L2.end
  measures "d205" distance of L0.end L1.end
  measures "d206" distance of L6.end L5.end
  measures "d207" distance of L5.end L4.end
  measures "d208" distance of L10.end L11.end
  measures "d209" distance of L9.end L10.end
  measures "d210" distance of L15.end L14.end
  measures "d211" distance of L14.end L13.end
extrude "Extrusion21" add sketch "Skizze21" against normal blind 25
sketch "Skizze22" plane through (0, 50, 0) normal (0, 1, 0) x (1, 0, 0)
  line L0 (-640, 975) -> (-640, 85) construction
  line L1 (-640, 85) -> (-640, 360) construction
  line L2 (-640, 85) -> (-365, 85) construction
  line L3 (-640, 360) -> (-640, 380) construction
  line L4 (-640, 380) -> (-640, 520) construction
  line L5 (-640, 520) -> (-640, 540) construction
  line L6 (-640, 540) -> (-640, 680) construction
  line L7 (-640, 680) -> (-640, 700) construction
  line L8 (-640, 360) -> (-645, 360)
  line L9 (-645, 360) -> (-645, 380)
  line L10 (-645, 380) -> (-640, 380)
  line L11 (-640, 380) -> (-640, 360)
  line L12 (-640, 520) -> (-645, 520)
  line L13 (-645, 520) -> (-645, 540)
  line L14 (-645, 540) -> (-640, 540)
  line L15 (-640, 540) -> (-640, 520)
  line L16 (-640, 680) -> (-645, 680)
  line L17 (-645, 680) -> (-645, 700)
  line L18 (-645, 700) -> (-640, 700)
  line L19 (-640, 700) -> (-640, 680)
  line L20 (-640, 85) -> (-830, 85) construction
  line L21 (-640, 85) -> (-830, 85) construction
  line L22 (-735, 85) -> (-735, 975) construction
  line L23 (-830, 975) -> (-640, 975) construction
  line L24 (-830, 360) -> (-830, 380) construction
  line L25 (-830, 520) -> (-830, 540) construction
  line L26 (-830, 680) -> (-830, 700) construction
  line L27 (-830, 360) -> (-825, 360)
  line L28 (-825, 360) -> (-825, 380)
  line L29 (-825, 380) -> (-830, 380)
  line L30 (-830, 380) -> (-830, 360)
  line L31 (-830, 520) -> (-825, 520)
  line L32 (-825, 520) -> (-825, 540)
  line L33 (-825, 540) -> (-830, 540)
  line L34 (-830, 540) -> (-830, 520)
  line L35 (-830, 680) -> (-825, 680)
  line L36 (-825, 680) -> (-825, 700)
  line L37 (-825, 700) -> (-830, 700)
  line L38 (-830, 700) -> (-830, 680)
  point P0 (0, 0)
  dimension "d217" = 275
  dimension "d218" = 90
  dimension "d219" = 20
  dimension "d220" = 140
  dimension "d221" = 20
  dimension "d222" = 180
  dimension "d223" = 140
  dimension "d224" = 180
  dimension "d225" = 20
  dimension "d226" = 5
  dimension "d227" = 20
  dimension "d228" = 5
  dimension "d229" = 20
  dimension "d230" = 5
  dimension "d231" = 20
  constraints: 72 end point, 15 symmetric about line, 6 parallel, 4 collinear, 4 horizontal, 4 perpendicular, 4 point on line, 2 midpoint
  measures "d217" distance of L0.end L1.end
  measures "d218" angle of L2 L1
  measures "d219" distance of L1.end L3.end
  measures "d220" distance of L3.end L4.end
  measures "d221" distance of L4.end L5.end
  measures "d222" angle of L5 L4
  measures "d223" distance of L5.end L6.end
  measures "d224" angle of L6 L5
  measures "d225" distance of L6.end L7.end
  measures "d226" distance of L9.end L10.end
  measures "d227" distance of L8.end L9.end
  measures "d228" distance of L13.end L14.end
  measures "d229" distance of L12.end L13.end
  measures "d230" distance of L17.end L18.end
  measures "d231" distance of L16.end L17.end
extrude "Extrusion22" add sketch "Skizze22" against normal blind 210
sketch "Skizze23" plane through (0, -160, 0) normal (0, -1, 0) x (1, 0, 0)
  line L0 (-830, -380) -> (-830, -360) projected
  line L1 (-640, -520) -> (-640, -380) projected
  line L2 (-830, -360) -> (-640, -360)
  line L3 (-640, -360) -> (-640, -380)
  line L4 (-640, -380) -> (-830, -380)
  line L5 (-830, -380) -> (-830, -360)
  line L6 (-830, -520) -> (-830, -540) projected
  line L7 (-640, -680) -> (-640, -540) projected
  line L8 (-830, -520) -> (-640, -520)
  line L9 (-640, -520) -> (-640, -540)
  line L10 (-640, -540) -> (-830, -540)
  line L11 (-830, -540) -> (-830, -520)
  line L12 (-830, -700) -> (-830, -680) projected
  line L13 (-640, -700) -> (-640, -680) projected
  line L14 (-830, -680) -> (-640, -680)
  line L15 (-640, -680) -> (-640, -700)
  line L16 (-640, -700) -> (-830, -700)
  line L17 (-830, -700) -> (-830, -680)
  point P0 (0, 0)
  constraints: 24 end point, 6 parallel, 3 horizontal, 3 perpendicular
extrude "Extrusion23" add sketch "Skizze23" along normal blind 5
sketch "Skizze24" plane through (-830, 0, -360) normal (0, 0, 1) x (1, 0, 0)
  line L0 (0, 0) -> (0, -165) projected
  line L1 (0, 0) -> (190, 0)
  line L2 (190, 0) -> (190, -20)
  line L3 (190, -20) -> (0, -20)
  line L4 (0, -20) -> (0, 0)
  line L5 (5, 50) -> (5, -160) construction
  line L6 (5, -160) -> (5, -110) construction
  line L7 (5, -160) -> (55, -160) construction
  line L8 (5, -110) -> (0, -110)
  line L9 (0, -110) -> (0, -90)
  line L10 (0, -90) -> (5, -90)
  line L11 (5, -90) -> (5, -110)
  line L12 (5, -110) -> (190, -110)
  line L13 (190, -110) -> (190, -90)
  line L14 (190, -90) -> (5, -90)
  line L15 (5, -90) -> (5, -110)
  point P0 (830, 0)
  dimension "d236" = 190
  dimension "d237" = 20
  dimension "d238" = 50
  dimension "d239" = 90
  dimension "d240" = 5
  dimension "d241" = 20
  dimension "d242" = 185
  dimension "d243" = 20
  constraints: 28 end point, 6 parallel, 4 horizontal, 4 perpendicular, 1 collinear
  measures "d236" distance of L2.end L3.end
  measures "d237" distance of L1.end L2.end
  measures "d238" distance of L5.end L6.end
  measures "d239" angle of L7 L6
  measures "d240" distance of L9.end L10.end
  measures "d241" distance of L8.end L9.end
  measures "d242" distance of L14.end L13.end
  measures "d243" distance of L13.end L12.end
extrude "Extrusion24" add sketch "Skizze24" along normal blind 5
sketch "Skizze25" plane through (-830, 0, -355) normal (0, 0, 1) x (1, 0, 0)
  line L0 (190, 0) -> (0, 0) projected
  line L1 (0, 0) -> (-5, 0)
  line L2 (-5, 0) -> (-5, -20)
  line L3 (-5, -20) -> (0, -20)
  line L4 (0, -20) -> (0, 0)
  line L5 (190, -20) -> (190, 0) projected
  line L6 (190, 0) -> (195, 0)
  line L7 (195, 0) -> (195, -20)
  line L8 (195, -20) -> (190, -20)
  line L9 (190, -20) -> (190, 0)
  line L10 (0, -110) -> (-5, -110)
  line L11 (-5, -110) -> (-5, -90)
  line L12 (-5, -90) -> (0, -90)
  line L13 (0, -90) -> (0, -110)
  line L14 (190, -110) -> (190, -90) projected
  line L15 (190, -90) -> (195, -90)
  line L16 (195, -90) -> (195, -110)
  line L17 (195, -110) -> (190, -110)
  line L18 (190, -110) -> (190, -90)
  point P0 (830, 0)
  dimension "d246" = 5
  dimension "d247" = 20
  dimension "d248" = 5
  dimension "d249" = 20
  dimension "d250" = 5
  dimension "d251" = 20
  dimension "d252" = 5
  dimension "d253" = 20
  constraints: 32 end point, 8 parallel, 4 horizontal, 4 perpendicular, 1 point on line
  measures "d246" distance of L3.end L2.end
  measures "d247" distance of L2.end L1.end
  measures "d248" distance of L7.end L8.end
  measures "d249" distance of L6.end L7.end
  measures "d250" distance of L11.end L12.end
  measures "d251" distance of L10.end L11.end
  measures "d252" distance of L16.end L17.end
  measures "d253" distance of L15.end L16.end
extrude "Extrusion25" add sketch "Skizze25" against normal blind 25
sketch "Skizze26" plane through (-640, 0, -700) normal (0, 0, -1) x (-1, 0, 0)
  line L0 (190, 0) -> (190, -165) projected
  line L1 (190, 0) -> (0, 0)
  line L2 (0, 0) -> (0, -20)
  line L3 (0, -20) -> (190, -20)
  line L4 (190, -20) -> (190, 0)
  line L5 (190, -165) -> (190, -110) construction
  line L6 (190, -165) -> (245, -165) construction
  line L7 (190, -110) -> (0, -110)
  line L8 (0, -110) -> (0, -90)
  line L9 (0, -90) -> (190, -90)
  line L10 (190, -90) -> (190, -110)
  point P0 (-640, 0)
  dimension "d256" = 190
  dimension "d257" = 20
  dimension "d258" = 55
  dimension "d259" = 90
  dimension "d260" = 190
  dimension "d261" = 20
  constraints: 20 end point, 4 parallel, 3 horizontal, 3 perpendicular, 1 vertical
  measures "d256" distance of L3.end L2.end
  measures "d257" distance of L2.end L1.end
  measures "d258" distance of L0.end L5.end
  measures "d259" angle of L6 L5
  measures "d260" distance of L8.end L9.end
  measures "d261" distance of L7.end L8.end
extrude "Extrusion26" add sketch "Skizze26" along normal blind 5
sketch "Skizze27" plane through (-640, 0, -705) normal (0, 0, -1) x (-1, 0, 0)
  line L0 (0, -20) -> (190, -20) projected
  line L1 (190, -20) -> (195, -20)
  line L2 (195, -20) -> (195, 0)
  line L3 (195, 0) -> (190, 0)
  line L4 (190, 0) -> (190, -20)
  line L5 (0, 0) -> (0, -20) projected
  line L6 (0, -20) -> (-5, -20)
  line L7 (-5, -20) -> (-5, 0)
  line L8 (-5, 0) -> (0, 0)
  line L9 (0, 0) -> (0, -20)
  line L10 (0, -110) -> (-5, -110)
  line L11 (-5, -110) -> (-5, -90)
  line L12 (-5, -90) -> (0, -90)
  line L13 (0, -90) -> (0, -110)
  line L14 (0, -110) -> (190, -110) projected
  line L15 (190, -110) -> (195, -110)
  line L16 (195, -110) -> (195, -90)
  line L17 (195, -90) -> (190, -90)
  line L18 (190, -90) -> (190, -110)
  point P0 (-640, 0)
  dimension "d264" = 5
  dimension "d265" = 20
  dimension "d266" = 5
  dimension "d267" = 20
  dimension "d268" = 5
  dimension "d269" = 20
  dimension "d270" = 5
  dimension "d271" = 20
  constraints: 32 end point, 8 parallel, 4 horizontal, 4 perpendicular
  measures "d264" distance of L3.end L2.end
  measures "d265" distance of L2.end L1.end
  measures "d266" distance of L7.end L8.end
  measures "d267" distance of L6.end L7.end
  measures "d268" distance of L11.end L12.end
  measures "d269" distance of L10.end L11.end
  measures "d270" distance of L17.end L16.end
  measures "d271" distance of L16.end L15.end
extrude "Extrusion27" add sketch "Skizze27" against normal blind 25
sketch "Skizze28" plane through (-880, 50, -5) normal (0, 0, 1) x (1, 0, 0)
  line L0 (25, -50) -> (235, -50) projected
  line L1 (25, -50) -> (25, -100)
  line L2 (25, -50) -> (25, -210) projected
  line L3 (25, -100) -> (75, -50)
  line L4 (0, -50) -> (25, -50) projected
  line L5 (75, -50) -> (25, -50)
  line L6 (235, -50) -> (185, -50)
  line L7 (50, -50) -> (240, -50) projected
  line L8 (235, -50) -> (285, -50) construction
  line L9 (185, -50) -> (235, -100)
  line L10 (235, -100) -> (235, -50)
  line L11 (235, 0) -> (235, -210) projected
  line L12 (1145, -50) -> (1145, -210) projected
  line L13 (1145, -50) -> (1145, -100)
  line L14 (1145, -50) -> (1195, -50) construction
  line L15 (1145, -100) -> (1095, -50)
  line L16 (935, -50) -> (1145, -50) projected
  line L17 (1095, -50) -> (1145, -50)
  line L18 (935, -50) -> (935, -210) projected
  line L19 (935, -50) -> (985, -50)
  line L20 (935, -50) -> (985, -50) construction
  line L21 (985, -50) -> (935, -100)
  line L22 (935, -100) -> (935, -50)
  line L23 (930, -50) -> (1120, -50) projected
  point P0 (880, -50)
  dimension "d274" = 50
  dimension "d275" = 45
  dimension "d276" = 50
  dimension "d277" = 180
  dimension "d278" = 45
  dimension "d279" = 50
  dimension "d280" = 90
  dimension "d281" = 315
  dimension "d282" = 50
  dimension "d283" = 0
  dimension "d284" = 45
  constraints: 30 end point, 4 perpendicular, 3 collinear, 3 equal length, 3 horizontal, 3 point on line
  measures "d274" distance of L0.start L1.end
  measures "d275" angle of L3 L1
  measures "d276" distance of L0.end L6.end
  measures "d277" angle of L6 L8
  measures "d278" angle of L9 L6
  measures "d279" distance of L12.start L13.end
  measures "d280" angle of L13 L14
  measures "d282" distance of L16.start L19.end
  measures "d283" distance between parallel lines of L19 L20
  measures "d284" angle of L19 L21
extrude "Extrusion28" add sketch "Skizze28" against normal blind 80
